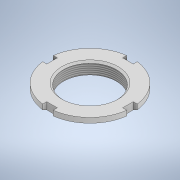
# Autodesk Inventor part: 69. Гайка стопорная
Saved by Autodesk Inventor 2021 (Build 250183000, 183)
## iProperties
Created: 2021-03-11
Part Number: 69. Гайка стопорная
Material: Типовые
Document SubType Name: Modeling
Designer: Данил
Density: 1 g/cm^3
Appearance: По умолчанию
Author: Данил
Autodesk Inventor part; units mm, degrees
ref_plane "YZ Plane" through (0, 0, 0) normal (1, 0, 0) x (0, 1, 0)
ref_plane "XZ Plane" through (0, 0, 0) normal (0, 1, 0) x (-1, 0, 0)
ref_plane "XY Plane" through (0, 0, 0) normal (0, 0, 1) x (1, 0, 0)
sketch "Эскиз1" plane through (0, 0, 0) normal (0, 0, 1) x (1, 0, 0)
  line L0 (0, 3.5) -> (0, -3.5)
  line L1 (15, -3.2113) -> (15.5, -3.5)
  line L2 (15.5, -3.5) -> (24, 0.6457)
  line L3 (15, -3.2113) -> (15, 2.5)
  line L4 (0, -3.5) -> (15.5, -3.5) construction
  line L5 (24, 0.6457) -> (24, 3.5)
  line L6 (24, 3.5) -> (16, 3.5)
  line L7 (15, 2.5) -> (16, 3.5)
  point P0 (0, 0)
  point P1 (0, 0)
  point P2 (15, 3.5)
  dimension "d0" = 7
  dimension "d1" = 60
  dimension "d2" = 31
  dimension "d3" = 30
  dimension "d4" = 26
  dimension "d5" = 48
  dimension "d9" = 1
  dimension "d10" = 45
  constraints: 16 end point, 3 vertical, 2 horizontal, 2 horizontal alignment, 2 point on line, 1 coincident, 1 midpoint
  measures "d0" distance of L0.start L0.end
  measures "d1" angle of L0 L1
  measures "d2" diameter of L1.end L0
  measures "d3" diameter of L3 L0
  measures "d4" angle of L4 L2
  measures "d5" diameter of L5 L0
  measures "d9" distance of L3.end point (15, 3.5)
  measures "d10" angle of L3 L7
revolve "Вращение1" add sketch "Эскиз1" angle 360 about axis through (0, 3.5, 0) along (0, -1, 0)
sketch "Эскиз2" plane through (0, 3.5, 0) normal (0, 1, 0) x (1, 0, 0)
  circle A0 centre (0, 0) radius 24 projected
  line L0 (3, 24) -> (-3, 24)
  line L1 (-3, 24) -> (-3, 21.5)
  line L2 (-3, 21.5) -> (3, 21.5)
  line L3 (3, 21.5) -> (3, 24)
  point P0 (0, 0)
  point P1 (0, 24)
  point P2 (3, 23.8118)
  point P3 (-3, 23.8118)
  dimension "d12" = 2.5
  dimension "d13" = 6
  constraints: 8 end point, 2 parallel, 1 horizontal, 1 midpoint, 1 perpendicular, 1 tangent, 1 vertical alignment
  measures "d12" distance of L0.end L1.end
  measures "d13" distance of L0.start L0.end
extrude "Выдавливание1" cut sketch "Эскиз2" against normal through all contours L3 L2 L1 A0 picked at (0, 22.3333)
pattern_circular "Круговой массив1" count 4 over 360 about axis through (0, -10, 0) along (0, 1, 0) of "Выдавливание1"
thread "Резьба1" size "M30x1" class "6H" standard "ISO Metric profile" length 20
